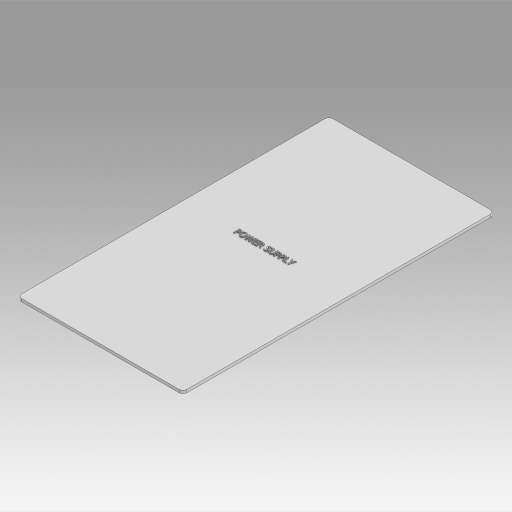
# Autodesk Inventor part: TOP_COVER
Saved by Autodesk Inventor 2023 (Build 270158000, 158)
## iProperties
Created: 2025-09-17
Part Number: TOP_COVER
Material: Generic
Document SubType Name: Modeling
Designer: NELLY NDUNG'U
Density: 1 g/cm^3
Appearance: Default
Author: NELLY NDUNG'U
Autodesk Inventor part; units mm, degrees
ref_plane "YZ Plane" through (0, 0, 0) normal (1, 0, 0) x (0, 1, 0)
ref_plane "XZ Plane" through (0, 0, 0) normal (0, 1, 0) x (-1, 0, 0)
ref_plane "XY Plane" through (0, 0, 0) normal (0, 0, 1) x (1, 0, 0)
sketch "Sketch1" plane through (0, 0, 0) normal (0, 1, 0) x (-1, 0, 0)
  line L0 (0, 0) -> (85, 0)
  line L1 (85, 0) -> (85, -160)
  line L2 (85, -160) -> (0, -160)
  line L3 (0, -160) -> (0, 0)
  dimension "d0" = 85
  dimension "d1" = 160
  constraints: 8 end point, 2 parallel, 1 horizontal, 1 perpendicular
  measures "d0" distance of L1.end L2.end
  measures "d1" distance of L0.end L1.end
extrude "Extrusion1" add sketch "Sketch1" along normal blind 1.5
fillet "Fillet1" radius 2 4 edges at (-85, 0.75, -160) (0, 0.75, -160) (-85, 0.75, 0) (0, 0.75, 0)
sketch "Sketch2" plane through (0, 0, 0) normal (0, -1, 0) x (1, 0, 0)
  arc A0 (0, -2) -> (-2, 0) centre (-2, -2) ccw projected
  line L0 (-83, 0) -> (-2, 0) projected
  arc A1 (-83, 0) -> (-85, -2) centre (-83, -2) ccw projected
  line L1 (-85, -158) -> (-85, -2) projected
  arc A2 (-85, -158) -> (-83, -160) centre (-83, -158) ccw projected
  line L2 (-2, -160) -> (-83, -160) projected
  arc A3 (-2, -160) -> (0, -158) centre (-2, -158) ccw projected
  line L3 (0, -2) -> (0, -158) projected
  line L4 (-82.5, -157.5) -> (-82.5, -2.5)
  line L5 (-82.5, -2.5) -> (-2.5, -2.5)
  line L6 (-2.5, -2.5) -> (-2.5, -157.5)
  line L7 (-2.5, -157.5) -> (-82.5, -157.5)
  line L8 (-81.75, -156.75) -> (-3.25, -156.75)
  line L9 (-3.25, -156.75) -> (-3.25, -3.25)
  line L10 (-3.25, -3.25) -> (-81.75, -3.25)
  line L11 (-81.75, -3.25) -> (-81.75, -156.75)
  point P0 (0, 0)
  dimension "d5" = 2.5
  dimension "d6" = 0.75
  constraints: 16 end point, 6 other
  measures "d5" distance between parallel lines of L2 L7
  measures "d6" distance between parallel lines of L7 L8
extrude "Extrusion2" cut sketch "Sketch2" against normal blind 0.75 contours L11 L10 L9 L8
extrude "Extrusion3" add sketch "Sketch2" along normal blind 0.75 contours L4 L5 L6 L7
sketch "Sketch3" plane through (0, 0.75, 0) normal (0, -1, 0) x (1, 0, 0)
  circle A0 centre (-15, -145) radius 2.5
  line L0 (-2, -160) -> (-83, -160) projected
  line L1 (0, -2) -> (0, -158) projected
  circle A1 centre (-15, -15) radius 2.5
  line L2 (-83, 0) -> (-2, 0) projected
  circle A2 centre (-70, -15) radius 2.5
  circle A3 centre (-70, -145) radius 2.5
  line L3 (-85, -158) -> (-85, -2) projected
  circle A4 centre (-15, -145) radius 0.5
  circle A5 centre (-70, -145) radius 0.5
  circle A6 centre (-70, -15) radius 0.5
  circle A7 centre (-15, -15) radius 0.5
  point P0 (0, 0)
  dimension "d11" = 5
  dimension "d12" = 15
  dimension "d13" = 15
  dimension "d14" = 5
  dimension "d15" = 15
  dimension "d16" = 15
  dimension "d17" = 5
  dimension "d18" = 5
  dimension "d19" = 15
  dimension "d20" = 15
  dimension "d21" = 15
  dimension "d22" = 15
  dimension "d23" = 2
  dimension "d24" = 2
  dimension "d25" = 2
  dimension "d26" = 2
  constraints: 8 centre point
  measures "d11" diameter of A0
  measures "d12" distance from line of A0.centre L0
  measures "d13" distance from line of A0.centre L1
  measures "d14" diameter of A1
  measures "d15" distance from line of A1.centre L2
  measures "d16" distance from line of A1.centre L1
  measures "d17" diameter of A2
  measures "d18" diameter of A3
  measures "d19" distance from line of A3.centre L3
  measures "d20" distance from line of A3.centre L0
  measures "d21" distance from line of L2 A2.centre
  measures "d22" distance from line of L3 A2.centre
  measures "d23" radial gap between concentric circles of A0 A4
  measures "d24" radial gap between concentric circles of A3 A5
  measures "d25" radial gap between concentric circles of A2 A6
  measures "d26" radial gap between concentric circles of A1 A7
extrude "Extrusion4" add sketch "Sketch3" along normal blind 0.75
sketch "Sketch4" plane through (0, 1.5, 0) normal (0, 1, 0) x (1, 0, 0)
  line L0 (-57.8038, 86.5831) -> (-28.2278, 86.5831) construction
  line L1 (-28.2278, 86.5831) -> (-28.2278, 83.4067) construction
  line L2 (-28.2278, 83.4067) -> (-57.8038, 83.4067) construction
  line L3 (-57.8038, 83.4067) -> (-57.8038, 86.5831) construction
  spline S0 degree 2 poles (-55.5684, 85.6001) (-55.5684, 85.4025) (-55.7092, 85.0468) (-55.8352, 84.9233) knots 0 0 0 1 2 2 2
  spline S1 degree 2 poles (-55.8352, 84.9233) (-55.9932, 84.7677) (-56.4206, 84.6071) (-56.7466, 84.6071) knots 0 0 0 1 2 2 2
  line L4 (-56.7466, 84.6071) -> (-57.0899, 84.6071)
  line L5 (-57.0899, 84.6071) -> (-57.0899, 83.4709)
  line L6 (-57.0899, 83.4709) -> (-57.495, 83.4709)
  line L7 (-57.495, 83.4709) -> (-57.495, 86.5189)
  line L8 (-57.495, 86.5189) -> (-56.7293, 86.5189)
  spline S2 degree 2 poles (-56.7293, 86.5189) (-56.4576, 86.5189) (-56.0772, 86.43) (-55.9315, 86.3287) knots 0 0 0 1 2 2 2
  spline S3 degree 2 poles (-55.9315, 86.3287) (-55.7611, 86.2126) (-55.5684, 85.8545) (-55.5684, 85.6001) knots 0 0 0 1 2 2 2
  spline S4 degree 2 poles (-55.9908, 85.5877) (-55.9908, 85.7458) (-56.0995, 85.978) (-56.2106, 86.0521) knots 0 0 0 1 2 2 2
  spline S5 degree 2 poles (-56.2106, 86.0521) (-56.3069, 86.1163) (-56.5638, 86.1682) (-56.754, 86.1682) knots 0 0 0 1 2 2 2
  line L9 (-56.754, 86.1682) -> (-57.0899, 86.1682)
  line L10 (-57.0899, 86.1682) -> (-57.0899, 84.9529)
  line L11 (-57.0899, 84.9529) -> (-56.8133, 84.9529)
  spline S6 degree 2 poles (-56.8133, 84.9529) (-56.5663, 84.9529) (-56.2625, 85.032) (-56.1637, 85.1357) knots 0 0 0 1 2 2 2
  spline S7 degree 2 poles (-56.1637, 85.1357) (-56.0723, 85.2271) (-55.9908, 85.442) (-55.9908, 85.5877) knots 0 0 0 1 2 2 2
  spline S8 degree 2 poles (-53.0268, 86.1706) (-52.8539, 85.9681) (-52.6612, 85.3753) (-52.6612, 84.9949) knots 0 0 0 1 2 2 2
  spline S9 degree 2 poles (-52.6612, 84.9949) (-52.6612, 84.6244) (-52.8489, 84.0242) (-53.0268, 83.8217) knots 0 0 0 1 2 2 2
  spline S10 degree 2 poles (-53.0268, 83.8217) (-53.2145, 83.6092) (-53.7109, 83.4067) (-54.0098, 83.4067) knots 0 0 0 1 2 2 2
  spline S11 degree 2 poles (-54.0098, 83.4067) (-54.3186, 83.4067) (-54.8126, 83.6167) (-54.9929, 83.8217) knots 0 0 0 1 2 2 2
  spline S12 degree 2 poles (-54.9929, 83.8217) (-55.1683, 84.0242) (-55.356, 84.6195) (-55.356, 84.9949) knots 0 0 0 1 2 2 2
  spline S13 degree 2 poles (-55.356, 84.9949) (-55.356, 85.3778) (-55.1658, 85.9607) (-54.9904, 86.1706) knots 0 0 0 1 2 2 2
  spline S14 degree 2 poles (-54.9904, 86.1706) (-54.8126, 86.3732) (-54.3161, 86.5831) (-54.0098, 86.5831) knots 0 0 0 1 2 2 2
  spline S15 degree 2 poles (-54.0098, 86.5831) (-53.6986, 86.5831) (-53.1997, 86.3658) (-53.0268, 86.1706) knots 0 0 0 1 2 2 2
  spline S16 degree 2 poles (-53.0836, 84.9949) (-53.0836, 85.2963) (-53.2145, 85.7631) (-53.333, 85.9162) knots 0 0 0 1 2 2 2
  spline S17 degree 2 poles (-53.333, 85.9162) (-53.4541, 86.0743) (-53.7949, 86.2324) (-54.0074, 86.2324) knots 0 0 0 1 2 2 2
  spline S18 degree 2 poles (-54.0074, 86.2324) (-54.2272, 86.2324) (-54.5582, 86.0793) (-54.6841, 85.9162) knots 0 0 0 1 2 2 2
  spline S19 degree 2 poles (-54.6841, 85.9162) (-54.8052, 85.7606) (-54.9336, 85.2913) (-54.9336, 84.9949) knots 0 0 0 1 2 2 2
  spline S20 degree 2 poles (-54.9336, 84.9949) (-54.9336, 84.3947) (-54.4297, 83.7574) (-54.0074, 83.7574) knots 0 0 0 1 2 2 2
  spline S21 degree 2 poles (-54.0074, 83.7574) (-53.585, 83.7574) (-53.0836, 84.3947) (-53.0836, 84.9949) knots 0 0 0 1 2 2 2
  line L12 (-48.8006, 86.5189) -> (-49.5663, 83.4709)
  line L13 (-49.5663, 83.4709) -> (-50.0207, 83.4709)
  line L14 (-50.0207, 83.4709) -> (-50.6407, 86.0002)
  line L15 (-50.6407, 86.0002) -> (-51.2434, 83.4709)
  line L16 (-51.2434, 83.4709) -> (-51.6929, 83.4709)
  line L17 (-51.6929, 83.4709) -> (-52.471, 86.5189)
  line L18 (-52.471, 86.5189) -> (-52.0536, 86.5189)
  line L19 (-52.0536, 86.5189) -> (-51.441, 83.9921)
  line L20 (-51.441, 83.9921) -> (-50.8334, 86.5189)
  line L21 (-50.8334, 86.5189) -> (-50.4209, 86.5189)
  line L22 (-50.4209, 86.5189) -> (-49.8083, 83.9625)
  line L23 (-49.8083, 83.9625) -> (-49.1982, 86.5189)
  line L24 (-49.1982, 86.5189) -> (-48.8006, 86.5189)
  line L25 (-48.4375, 83.4709) -> (-48.4375, 86.5189)
  line L26 (-48.4375, 86.5189) -> (-46.5306, 86.5189)
  line L27 (-46.5306, 86.5189) -> (-46.5306, 86.1583)
  line L28 (-46.5306, 86.1583) -> (-48.0324, 86.1583)
  line L29 (-48.0324, 86.1583) -> (-48.0324, 85.3234)
  line L30 (-48.0324, 85.3234) -> (-46.6319, 85.3234)
  line L31 (-46.6319, 85.3234) -> (-46.6319, 84.9628)
  line L32 (-46.6319, 84.9628) -> (-48.0324, 84.9628)
  line L33 (-48.0324, 84.9628) -> (-48.0324, 83.8315)
  line L34 (-48.0324, 83.8315) -> (-46.5306, 83.8315)
  line L35 (-46.5306, 83.8315) -> (-46.5306, 83.4709)
  line L36 (-46.5306, 83.4709) -> (-48.4375, 83.4709)
  line L37 (-43.7271, 83.4709) -> (-44.2533, 83.4709)
  line L38 (-44.2533, 83.4709) -> (-45.2166, 84.6837)
  line L39 (-45.2166, 84.6837) -> (-45.6809, 84.6837)
  line L40 (-45.6809, 84.6837) -> (-45.6809, 83.4709)
  line L41 (-45.6809, 83.4709) -> (-46.086, 83.4709)
  line L42 (-46.086, 83.4709) -> (-46.086, 86.5189)
  line L43 (-46.086, 86.5189) -> (-45.3005, 86.5189)
  spline S22 degree 2 poles (-45.3005, 86.5189) (-45.0387, 86.5189) (-44.6855, 86.4621) (-44.525, 86.3584) knots 0 0 0 1 2 2 2
  spline S23 degree 2 poles (-44.525, 86.3584) (-44.3644, 86.2546) (-44.1792, 85.9311) (-44.1792, 85.6915) knots 0 0 0 1 2 2 2
  spline S24 degree 2 poles (-44.1792, 85.6915) (-44.1792, 85.358) (-44.52, 84.906) (-44.8115, 84.7973) knots 0 0 0 1 2 2 2
  line L44 (-44.8115, 84.7973) -> (-43.7271, 83.4709)
  spline S25 degree 2 poles (-44.6015, 85.6594) (-44.6015, 85.7927) (-44.6954, 85.9977) (-44.7942, 86.0644) knots 0 0 0 1 2 2 2
  spline S26 degree 2 poles (-44.7942, 86.0644) (-44.8806, 86.1212) (-45.1104, 86.1682) (-45.2783, 86.1682) knots 0 0 0 1 2 2 2
  line L45 (-45.2783, 86.1682) -> (-45.6809, 86.1682)
  line L46 (-45.6809, 86.1682) -> (-45.6809, 85.0221)
  line L47 (-45.6809, 85.0221) -> (-45.3252, 85.0221)
  spline S27 degree 2 poles (-45.3252, 85.0221) (-45.1499, 85.0221) (-44.8708, 85.0838) (-44.7744, 85.1802) knots 0 0 0 1 2 2 2
  spline S28 degree 2 poles (-44.7744, 85.1802) (-44.6855, 85.2642) (-44.6015, 85.5013) (-44.6015, 85.6594) knots 0 0 0 1 2 2 2
  spline S29 degree 2 poles (-41.3263, 83.4166) (-41.6573, 83.4166) (-42.1216, 83.5549) (-42.3266, 83.6537) knots 0 0 0 1 2 2 2
  line L48 (-42.3266, 83.6537) -> (-42.3266, 84.1625)
  line L49 (-42.3266, 84.1625) -> (-42.297, 84.1625)
  spline S30 degree 2 poles (-42.297, 84.1625) (-42.0969, 83.9748) (-41.5906, 83.7673) (-41.3559, 83.7673) knots 0 0 0 1 2 2 2
  spline S31 degree 2 poles (-41.3559, 83.7673) (-41.02, 83.7673) (-40.6767, 84.0464) (-40.6767, 84.2761) knots 0 0 0 1 2 2 2
  spline S32 degree 2 poles (-40.6767, 84.2761) (-40.6767, 84.4589) (-40.857, 84.6862) (-41.0521, 84.743) knots 0 0 0 1 2 2 2
  spline S33 degree 2 poles (-41.0521, 84.743) (-41.1929, 84.7825) (-41.4276, 84.8368) (-41.6029, 84.8813) knots 0 0 0 1 2 2 2
  spline S34 degree 2 poles (-41.6029, 84.8813) (-41.761, 84.9233) (-42.0105, 85.0493) (-42.1068, 85.1505) knots 0 0 0 1 2 2 2
  spline S35 degree 2 poles (-42.1068, 85.1505) (-42.2007, 85.2518) (-42.3044, 85.5235) (-42.3044, 85.7013) knots 0 0 0 1 2 2 2
  spline S36 degree 2 poles (-42.3044, 85.7013) (-42.3044, 86.0718) (-41.7264, 86.5733) (-41.2794, 86.5733) knots 0 0 0 1 2 2 2
  spline S37 degree 2 poles (-41.2794, 86.5733) (-41.0225, 86.5733) (-40.568, 86.472) (-40.3729, 86.3757) knots 0 0 0 1 2 2 2
  line L50 (-40.3729, 86.3757) -> (-40.3729, 85.8915)
  line L51 (-40.3729, 85.8915) -> (-40.4025, 85.8915)
  spline S38 degree 2 poles (-40.4025, 85.8915) (-40.5482, 86.0249) (-41.0027, 86.2225) (-41.2522, 86.2225) knots 0 0 0 1 2 2 2
  spline S39 degree 2 poles (-41.2522, 86.2225) (-41.5338, 86.2225) (-41.882, 85.9582) (-41.882, 85.7433) knots 0 0 0 1 2 2 2
  spline S40 degree 2 poles (-41.882, 85.7433) (-41.882, 85.5507) (-41.677, 85.321) (-41.4844, 85.2691) knots 0 0 0 1 2 2 2
  spline S41 degree 2 poles (-41.4844, 85.2691) (-41.3559, 85.2345) (-40.983, 85.1456) (-40.8595, 85.1085) knots 0 0 0 1 2 2 2
  spline S42 degree 2 poles (-40.8595, 85.1085) (-40.5458, 85.0122) (-40.2543, 84.6244) (-40.2543, 84.3404) knots 0 0 0 1 2 2 2
  spline S43 degree 2 poles (-40.2543, 84.3404) (-40.2543, 84.1601) (-40.4, 83.8143) (-40.5309, 83.6932) knots 0 0 0 1 2 2 2
  spline S44 degree 2 poles (-40.5309, 83.6932) (-40.6767, 83.5598) (-41.0472, 83.4166) (-41.3263, 83.4166) knots 0 0 0 1 2 2 2
  spline S45 degree 2 poles (-38.7772, 83.4067) (-39.0465, 83.4067) (-39.4466, 83.5475) (-39.5874, 83.6883) knots 0 0 0 1 2 2 2
  spline S46 degree 2 poles (-39.5874, 83.6883) (-39.7479, 83.8464) (-39.8789, 84.291) (-39.8789, 84.617) knots 0 0 0 1 2 2 2
  line L52 (-39.8789, 84.617) -> (-39.8789, 86.5189)
  line L53 (-39.8789, 86.5189) -> (-39.4738, 86.5189)
  line L54 (-39.4738, 86.5189) -> (-39.4738, 84.617)
  spline S47 degree 2 poles (-39.4738, 84.617) (-39.4738, 84.4046) (-39.4194, 84.1181) (-39.3429, 84.002) knots 0 0 0 1 2 2 2
  spline S48 degree 2 poles (-39.3429, 84.002) (-39.2614, 83.8785) (-38.9798, 83.7525) (-38.7772, 83.7525) knots 0 0 0 1 2 2 2
  spline S49 degree 2 poles (-38.7772, 83.7525) (-38.587, 83.7525) (-38.2906, 83.8785) (-38.2091, 84.002) knots 0 0 0 1 2 2 2
  spline S50 degree 2 poles (-38.2091, 84.002) (-38.1326, 84.1181) (-38.0782, 84.4021) (-38.0782, 84.6071) knots 0 0 0 1 2 2 2
  line L55 (-38.0782, 84.6071) -> (-38.0782, 86.5189)
  line L56 (-38.0782, 86.5189) -> (-37.6731, 86.5189)
  line L57 (-37.6731, 86.5189) -> (-37.6731, 84.617)
  spline S51 degree 2 poles (-37.6731, 84.617) (-37.6731, 84.2984) (-37.8016, 83.8439) (-37.9646, 83.6883) knots 0 0 0 1 2 2 2
  spline S52 degree 2 poles (-37.9646, 83.6883) (-38.1103, 83.545) (-38.4956, 83.4067) (-38.7772, 83.4067) knots 0 0 0 1 2 2 2
  spline S53 degree 2 poles (-35.1661, 85.6001) (-35.1661, 85.4025) (-35.3069, 85.0468) (-35.4328, 84.9233) knots 0 0 0 1 2 2 2
  spline S54 degree 2 poles (-35.4328, 84.9233) (-35.5909, 84.7677) (-36.0182, 84.6071) (-36.3443, 84.6071) knots 0 0 0 1 2 2 2
  line L58 (-36.3443, 84.6071) -> (-36.6876, 84.6071)
  line L59 (-36.6876, 84.6071) -> (-36.6876, 83.4709)
  line L60 (-36.6876, 83.4709) -> (-37.0927, 83.4709)
  line L61 (-37.0927, 83.4709) -> (-37.0927, 86.5189)
  line L62 (-37.0927, 86.5189) -> (-36.327, 86.5189)
  spline S55 degree 2 poles (-36.327, 86.5189) (-36.0553, 86.5189) (-35.6749, 86.43) (-35.5292, 86.3287) knots 0 0 0 1 2 2 2
  spline S56 degree 2 poles (-35.5292, 86.3287) (-35.3587, 86.2126) (-35.1661, 85.8545) (-35.1661, 85.6001) knots 0 0 0 1 2 2 2
  spline S57 degree 2 poles (-35.5884, 85.5877) (-35.5884, 85.7458) (-35.6971, 85.978) (-35.8083, 86.0521) knots 0 0 0 1 2 2 2
  spline S58 degree 2 poles (-35.8083, 86.0521) (-35.9046, 86.1163) (-36.1615, 86.1682) (-36.3517, 86.1682) knots 0 0 0 1 2 2 2
  line L63 (-36.3517, 86.1682) -> (-36.6876, 86.1682)
  line L64 (-36.6876, 86.1682) -> (-36.6876, 84.9529)
  line L65 (-36.6876, 84.9529) -> (-36.411, 84.9529)
  spline S59 degree 2 poles (-36.411, 84.9529) (-36.164, 84.9529) (-35.8601, 85.032) (-35.7613, 85.1357) knots 0 0 0 1 2 2 2
  spline S60 degree 2 poles (-35.7613, 85.1357) (-35.6699, 85.2271) (-35.5884, 85.442) (-35.5884, 85.5877) knots 0 0 0 1 2 2 2
  spline S61 degree 2 poles (-32.8541, 85.6001) (-32.8541, 85.4025) (-32.9949, 85.0468) (-33.1209, 84.9233) knots 0 0 0 1 2 2 2
  spline S62 degree 2 poles (-33.1209, 84.9233) (-33.279, 84.7677) (-33.7063, 84.6071) (-34.0323, 84.6071) knots 0 0 0 1 2 2 2
  line L66 (-34.0323, 84.6071) -> (-34.3757, 84.6071)
  line L67 (-34.3757, 84.6071) -> (-34.3757, 83.4709)
  line L68 (-34.3757, 83.4709) -> (-34.7807, 83.4709)
  line L69 (-34.7807, 83.4709) -> (-34.7807, 86.5189)
  line L70 (-34.7807, 86.5189) -> (-34.015, 86.5189)
  spline S63 degree 2 poles (-34.015, 86.5189) (-33.7433, 86.5189) (-33.363, 86.43) (-33.2172, 86.3287) knots 0 0 0 1 2 2 2
  spline S64 degree 2 poles (-33.2172, 86.3287) (-33.0468, 86.2126) (-32.8541, 85.8545) (-32.8541, 85.6001) knots 0 0 0 1 2 2 2
  spline S65 degree 2 poles (-33.2765, 85.5877) (-33.2765, 85.7458) (-33.3852, 85.978) (-33.4963, 86.0521) knots 0 0 0 1 2 2 2
  spline S66 degree 2 poles (-33.4963, 86.0521) (-33.5927, 86.1163) (-33.8495, 86.1682) (-34.0397, 86.1682) knots 0 0 0 1 2 2 2
  line L71 (-34.0397, 86.1682) -> (-34.3757, 86.1682)
  line L72 (-34.3757, 86.1682) -> (-34.3757, 84.9529)
  line L73 (-34.3757, 84.9529) -> (-34.099, 84.9529)
  spline S67 degree 2 poles (-34.099, 84.9529) (-33.852, 84.9529) (-33.5482, 85.032) (-33.4494, 85.1357) knots 0 0 0 1 2 2 2
  spline S68 degree 2 poles (-33.4494, 85.1357) (-33.358, 85.2271) (-33.2765, 85.442) (-33.2765, 85.5877) knots 0 0 0 1 2 2 2
  line L74 (-30.7027, 83.4709) -> (-32.4688, 83.4709)
  line L75 (-32.4688, 83.4709) -> (-32.4688, 86.5189)
  line L76 (-32.4688, 86.5189) -> (-32.0637, 86.5189)
  line L77 (-32.0637, 86.5189) -> (-32.0637, 83.8315)
  line L78 (-32.0637, 83.8315) -> (-30.7027, 83.8315)
  line L79 (-30.7027, 83.8315) -> (-30.7027, 83.4709)
  line L80 (-28.25, 86.5189) -> (-29.28, 84.8195)
  line L81 (-29.28, 84.8195) -> (-29.28, 83.4709)
  line L82 (-29.28, 83.4709) -> (-29.6851, 83.4709)
  line L83 (-29.6851, 83.4709) -> (-29.6851, 84.7776)
  line L84 (-29.6851, 84.7776) -> (-30.7151, 86.5189)
  line L85 (-30.7151, 86.5189) -> (-30.2656, 86.5189)
  line L86 (-30.2656, 86.5189) -> (-29.4776, 85.1777)
  line L87 (-29.4776, 85.1777) -> (-28.6798, 86.5189)
  line L88 (-28.6798, 86.5189) -> (-28.25, 86.5189)
  point P0 (0, 0)
  constraints: 2 other
emboss "Emboss1" sketch "Sketch4" operation add depth 0.5 direction (0, -1, 0)
body "Solid1"
